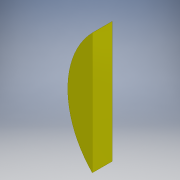
# Autodesk Inventor part: frameMount
Saved by Autodesk Inventor 2016 (Build 200138000, 138)
## iProperties
Created: 2015-11-15
Part Number: frameMount
Material: ABS Plastic
Document SubType Name: Modeling
Designer: Artur
Density: 1.06 g/cm^3
Appearance: Smooth - White
Mass: 9.43199 g
Surface Area: 33.2764 cm^2
Volume: 8.89811 cm^3
Author: Artur
Autodesk Inventor part; units mm, degrees
ref_plane "YZ Plane" through (0, 0, 0) normal (1, 0, 0) x (0, 1, 0)
ref_plane "XZ Plane" through (0, 0, 0) normal (0, 1, 0) x (-1, 0, 0)
ref_plane "XY Plane" through (0, 0, 0) normal (0, 0, 1) x (1, 0, 0)
sketch "Sketch1" plane through (0, 0, 0) normal (0, 1, 0) x (-1, 0, 0)
  line L0 (0, 0) -> (0, -73)
  arc A0 (0, -73) -> (0, 0) centre (-37.7359, -36.5) ccw
  dimension "d0" = 73
  dimension "d2" = 52.5
  constraints: 2 end point, 2 point on circle, 1 centre point, 1 coincident, 1 vertical
  measures "d0" distance of L0.start L0.end
  measures "d2" radius of A0
extrude "Extrusion1" add sketch "Sketch1" along normal blind 12
body "Solid1"
